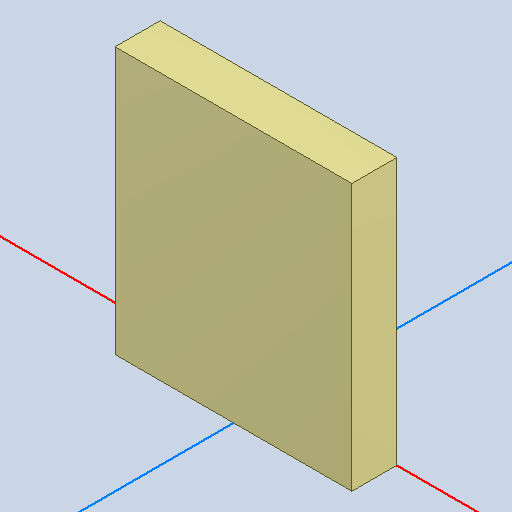
# Autodesk Inventor part: LED5MM
Saved by Autodesk Inventor 2022 (Build 260153000, 153)
## iProperties
Created: 2023-03-06
Part Number: LED5MM
Material: Типовые
Document SubType Name: Modeling
Designer: Иван Петров
Density: 1 g/cm^3
Appearance: LED5MM, LED5MM
Author: Иван Петров
Autodesk Inventor part; units mm, degrees
ref_plane "YZ Plane" through (0, 0, 0) normal (1, 0, 0) x (0, 1, 0)
ref_plane "XZ Plane" through (0, 0, 0) normal (0, 1, 0) x (-1, 0, 0)
ref_plane "XY Plane" through (0, 0, 0) normal (0, 0, 1) x (1, 0, 0)
sketch "LED5MM, LED5MM_8" plane through (0, 0, 0) normal (0, 0, 1) x (1, 0, 0)
  line L0 (-2.6162, 3.302) -> (2.6416, 3.302)
  line L1 (2.6416, 3.302) -> (2.6416, -2.6162)
  line L2 (2.6416, -2.6162) -> (-2.6162, -2.6162)
  line L3 (-2.6162, -2.6162) -> (-2.6162, 3.302)
  constraints: 8 end point
extrude "Выдавливание1" add sketch "LED5MM, LED5MM_8" along normal blind 1
